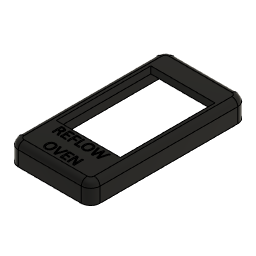
LCD Cover v3 (Autodesk Fusion 360 design; units mm, degrees)
Autodesk Fusion 360 part; units mm, degrees
(part 1 of 2)
sketch "Sketch1" plane through (0, 0, 0) normal (0, 0, 1) x (1, 0, 0)
  line L0 (27, -64) -> (-27, -64)
  line L1 (-32, -59) -> (-32, 59)
  line L2 (-27, 64) -> (27, 64)
  line L3 (32, 59) -> (32, -59)
  line L4 (32, -64) -> (-32, 64) construction
  line L5 (-32, -64) -> (32, 64) construction
  arc A0 (-27, 64) -> (-32, 59) centre (-27, 59) ccw
  arc A1 (32, 59) -> (27, 64) centre (27, 59) ccw
  arc A2 (-32, -59) -> (-27, -64) centre (-27, -59) ccw
  arc A3 (27, -64) -> (32, -59) centre (27, -59) ccw
  arc A4 (27, -67) -> (35, -59) centre (27, -59) ccw
  line L6 (35, 59) -> (35, -59)
  arc A5 (35, 59) -> (27, 67) centre (27, 59) ccw
  line L7 (-27, 67) -> (27, 67)
  arc A6 (-27, 67) -> (-35, 59) centre (-27, 59) ccw
  line L8 (-35, -59) -> (-35, 59)
  arc A7 (-35, -59) -> (-27, -67) centre (-27, -59) ccw
  line L9 (27, -67) -> (-27, -67)
  line L10 (24.75, 56.35) -> (-24.75, 56.35) construction
  line L11 (-24.75, 56.35) -> (-24.75, -37.75) construction
  line L12 (-24.75, -37.75) -> (24.75, -37.75) construction
  line L13 (24.75, -37.75) -> (24.75, 56.35) construction
  line L14 (24.75, 56.35) -> (-24.75, -37.75) construction
  line L15 (-24.75, 56.35) -> (24.75, -37.75) construction
  line L16 (0, 0) -> (0, 9.3) construction
  line L17 (24.48, 44) -> (-24.48, 44)
  line L18 (-24.48, 44) -> (-24.48, -31)
  line L19 (-24.48, -31) -> (24.48, -31)
  line L20 (24.48, -31) -> (24.48, 44)
  line L21 (24.48, 44) -> (-24.48, -31) construction
  line L22 (-24.48, 44) -> (24.48, -31) construction
  point P0 (0, 9.3)
  point P1 (0, 6.5)
  dimension "d1" = 64
  dimension "d2" = 128
  dimension "d3" = 5
  dimension "d4" = 5
  dimension "d5" = 5
  dimension "d6" = 5
  dimension "d7" = -3
  dimension "d8" = 49.5
  dimension "d9" = 94.1
  dimension "d11" = 54.7
  dimension "d12" = 48.96
  dimension "d13" = 75
  dimension "d14" = 12.35
  dimension "d24" = 15.56
  dimension "d25" = 39
  constraint horizontal L0
  constraint perpendicular L0 L1
  constraint parallel L0 L2
  constraint parallel L1 L3
  constraint coincident L4 L16.start
  constraint coincident L5 L16.start
  constraint coincident L16.start origin
  constraint coincident L4.end L1
  constraint coincident L4.end L2
  constraint tangent L1 A0
  constraint tangent L2 A0
  constraint coincident L5.end L2
  constraint coincident L5.end L3
  constraint tangent L2 A1
  constraint tangent L3 A1
  constraint coincident L5.start L1
  constraint coincident L5.start L0
  constraint tangent L1 A2
  constraint tangent L0 A2
  constraint coincident L4.start L0
  constraint coincident L4.start L3
  constraint tangent L0 A3
  constraint tangent L3 A3
  constraint horizontal L10
  constraint perpendicular L10 L11
  constraint parallel L10 L12
  constraint parallel L11 L13
  constraint coincident L14 P0
  constraint coincident L15 P0
  constraint coincident P0 L16.end
  constraint vertical L16
  constraint horizontal L17
  constraint perpendicular L17 L18
  constraint parallel L17 L19
  constraint parallel L18 L20
  constraint coincident L21 P1
  constraint coincident L22 P1
  constraint coincident L16 P1
  measures "d1" distance of L4.end L5.end
  measures "d2" distance of L5.start L4.end
  measures "d3" radius of A0
  measures "d4" radius of A1
  measures "d5" radius of A2
  measures "d6" radius of A3
  measures "d8" distance of L11.end L12.end
  measures "d9" distance of L10.end L11.end
  measures "d11" distance of L2 P0
  measures "d12" distance of L18.end L19.end
  measures "d13" distance of L17.end L18.end
  measures "d14" distance of L10 L17
extrude "Extrude1" add sketch "Sketch1" against normal blind 14.7 contours A4 L6 A5 L7 A6 L8 A7 L9
extrude "Extrude2" add sketch "Sketch1" along normal blind 3 contours L0 L1 L2 L3 A0 A1 A2 A3 | A4 L6 A5 L7 A6 L8 A7 L9
chamfer "Chamfer1" distance 3 angle 45 4 edges at (-24.48, 6.5, 3) (0, 44, 3) (24.48, 6.5, 3) (0, -31, 3)
fillet "Fillet1" radius 5 8 edges at (35, 0, 3) (32.6569, 64.6569, 3) (0, 67, 3) (-32.6569, 64.6569, 3) (-35, 0, 3) (-32.6569, -64.6569, 3) (0, -67, 3) (32.6569, -64.6569, 3)
fillet "Fillet2" radius 2 8 edges at (-32, 0, 0) (-30.5355, 62.5355, 0) (0, 64, 0) (30.5355, 62.5355, 0) (32, 0, 0) (30.5355, -62.5355, 0) (0, -64, 0) (-30.5355, -62.5355, 0)
sketch "Sketch2" plane through (0, 0, 3) normal (0, 0, 1) x (-1, 0, 0)
  line L0 (-27.48, -47) -> (-27.48, 34)
  line L1 (-27.48, 34) -> (27.48, 34)
  line L2 (27.48, 34) -> (27.48, -47)
  line L3 (27.48, -47) -> (-27.48, -47)
  line L4 (-30, 59) -> (-30, -59)
  arc A0 (-30, -59) -> (-27, -62) centre (-27, -59) ccw
  line L5 (-27, -62) -> (27, -62)
  arc A1 (27, -62) -> (30, -59) centre (27, -59) ccw
  line L6 (30, -59) -> (30, 59)
  arc A2 (30, 59) -> (27, 62) centre (27, 59) ccw
  line L7 (27, 62) -> (-27, 62)
  arc A3 (-27, 62) -> (-30, 59) centre (-27, 59) ccw
  line L8 (27.48, 34) -> (30, 34) construction
  line L9 (-27.48, 34) -> (-30, 34) construction
  line L10 (-30, 34) -> (29.1213, 61.1213) construction
  line L11 (30, 34) -> (-29.1213, 61.1213) construction
  line L12 (-1, 47.2622) -> (1, 47.2622) construction
  line L13 (1, 47.2622) -> (1, 48.2622) construction
  line L14 (1, 48.2622) -> (-1, 48.2622) construction
  line L15 (-1, 48.2622) -> (-1, 47.2622) construction
  line L16 (-1, 47.2622) -> (1, 48.2622) construction
  line L17 (1, 47.2622) -> (-1, 48.2622) construction
  spline S0 degree 3 poles (15.5846, 43.9099) (15.5852, 43.9255) (15.5864, 43.9553) (15.5977, 43.9829) (15.6031, 43.996) knots 0 0 0 0 0.004638 0.008871 0.008871 0.008871 0.008871
  spline S1 degree 3 poles (15.6031, 43.996) (15.6121, 44.0082) (15.6328, 44.0362) (15.6649, 44.0499) (15.6831, 44.0576) knots 0 0 0 0 0.004472 0.010255 0.010255 0.010255 0.010255
  spline S2 degree 3 poles (15.6831, 44.0576) (15.7075, 44.0655) (15.7637, 44.0836) (15.8223, 44.0906) (15.8554, 44.0945) knots 0 0 0 0 0.007692 0.017658 0.017658 0.017658 0.017658
  spline S3 degree 3 poles (15.8554, 44.0945) (15.8984, 44.0981) (15.9967, 44.1062) (16.0953, 44.1066) (16.1508, 44.1068) knots 0 0 0 0 0.012956 0.029574 0.029574 0.029574 0.029574
  spline S4 degree 3 poles (16.1508, 44.1068) (16.1993, 44.1066) (16.2866, 44.1061) (16.3736, 44.0981) (16.4123, 44.0945) knots 0 0 0 0 0.014542 0.026194 0.026194 0.026194 0.026194
  spline S5 degree 3 poles (16.4123, 44.0945) (16.4431, 44.0903) (16.499, 44.0828) (16.5517, 44.0633) (16.5754, 44.0545) knots 0 0 0 0 0.009295 0.016836 0.016836 0.016836 0.016836
  spline S6 degree 3 poles (16.5754, 44.0545) (16.5945, 44.0447) (16.6317, 44.0256) (16.658, 43.9932) (16.6708, 43.9776) knots 0 0 0 0 0.006385 0.012372 0.012372 0.012372 0.012372
  spline S7 degree 3 poles (16.6708, 43.9776) (16.6819, 43.9594) (16.7058, 43.9205) (16.7211, 43.8775) (16.7292, 43.8545) knots 0 0 0 0 0.006373 0.013658 0.013658 0.013658 0.013658
  line L18 (16.7292, 43.8545) -> (17.4615, 41.9776)
  spline S8 degree 3 poles (17.4615, 41.9776) (17.5042, 41.8747) (17.5866, 41.6757) (17.6828, 41.483) (17.7292, 41.3899) knots 0 0 0 0 0.033392 0.064596 0.064596 0.064596 0.064596
  spline S9 degree 3 poles (17.7292, 41.3899) (17.7767, 41.3046) (17.8692, 41.1384) (17.9965, 40.9972) (18.0585, 40.9284) knots 0 0 0 0 0.029168 0.056854 0.056854 0.056854 0.056854
  spline S10 degree 3 poles (18.0585, 40.9284) (18.1252, 40.8672) (18.2597, 40.744) (18.4246, 40.6661) (18.5077, 40.6268) knots 0 0 0 0 0.026986 0.05438 0.05438 0.05438 0.05438
  spline S11 degree 3 poles (18.5077, 40.6268) (18.6018, 40.5954) (18.8033, 40.5282) (19.0159, 40.5223) (19.1292, 40.5191) knots 0 0 0 0 0.029585 0.063385 0.063385 0.063385 0.063385
  line L19 (19.1292, 40.5191) -> (19.8369, 40.5191)
  line L20 (19.8369, 40.5191) -> (19.8369, 43.9099)
  spline S12 degree 3 poles (19.8369, 43.9099) (19.838, 43.9257) (19.8401, 43.9567) (19.8565, 43.9831) (19.8646, 43.996) knots 0 0 0 0 0.004667 0.009174 0.009174 0.009174 0.009174
  spline S13 degree 3 poles (19.8646, 43.996) (19.8758, 44.008) (19.9001, 44.0338) (19.933, 44.0473) (19.9508, 44.0545) knots 0 0 0 0 0.004844 0.01052 0.01052 0.01052 0.01052
  spline S14 degree 3 poles (19.9508, 44.0545) (19.9737, 44.0617) (20.0261, 44.078) (20.0803, 44.0866) (20.1108, 44.0914) knots 0 0 0 0 0.007206 0.01644 0.01644 0.01644 0.01644
  spline S15 degree 3 poles (20.1108, 44.0914) (20.1489, 44.0959) (20.2338, 44.1059) (20.3192, 44.1065) (20.3662, 44.1068) knots 0 0 0 0 0.01152 0.025602 0.025602 0.025602 0.025602
  spline S16 degree 3 poles (20.3662, 44.1068) (20.4131, 44.1065) (20.4986, 44.1059) (20.5834, 44.0959) (20.6215, 44.0914) knots 0 0 0 0 0.014082 0.025602 0.025602 0.025602 0.025602
  spline S17 degree 3 poles (20.6215, 44.0914) (20.6522, 44.0865) (20.7074, 44.0778) (20.7609, 44.0617) (20.7846, 44.0545) knots 0 0 0 0 0.009309 0.016737 0.016737 0.016737 0.016737
  spline S18 degree 3 poles (20.7846, 44.0545) (20.803, 44.0475) (20.8365, 44.0346) (20.8601, 44.008) (20.8708, 43.996) knots 0 0 0 0 0.005814 0.010547 0.010547 0.010547 0.010547
  spline S19 degree 3 poles (20.8708, 43.996) (20.8779, 43.983) (20.8927, 43.9562) (20.8945, 43.9256) (20.8954, 43.9099) knots 0 0 0 0 0.004406 0.009062 0.009062 0.009062 0.009062
  line L21 (20.8954, 43.9099) -> (20.8954, 36.5376)
  spline S20 degree 3 poles (20.8954, 36.5376) (20.8932, 36.4662) (20.8892, 36.3389) (20.8059, 36.244) (20.7692, 36.2022) knots 0 0 0 0 0.020627 0.03683 0.03683 0.03683 0.03683
  spline S21 degree 3 poles (20.7692, 36.2022) (20.7273, 36.1744) (20.6458, 36.1204) (20.5487, 36.1112) (20.5015, 36.1068) knots 0 0 0 0 0.014839 0.028813 0.028813 0.028813 0.028813
  line L22 (20.5015, 36.1068) -> (18.8092, 36.1068)
  spline S22 degree 3 poles (18.8092, 36.1068) (18.7171, 36.1072) (18.5498, 36.1078) (18.3828, 36.1177) (18.3077, 36.1222) knots 0 0 0 0 0.027618 0.050186 0.050186 0.050186 0.050186
  spline S23 degree 3 poles (18.3077, 36.1222) (18.2443, 36.1273) (18.1242, 36.1369) (18.0043, 36.1499) (17.9477, 36.156) knots 0 0 0 0 0.019068 0.03616 0.03616 0.03616 0.03616
  spline S24 degree 3 poles (17.9477, 36.156) (17.8012, 36.1852) (17.5205, 36.241) (17.2579, 36.3542) (17.1323, 36.4084) knots 0 0 0 0 0.044667 0.085564 0.085564 0.085564 0.085564
  spline S25 degree 3 poles (17.1323, 36.4084) (17.0202, 36.4685) (16.8013, 36.5858) (16.6246, 36.7602) (16.5385, 36.8453) knots 0 0 0 0 0.037954 0.074067 0.074067 0.074067 0.074067
  spline S26 degree 3 poles (16.5385, 36.8453) (16.4634, 36.9369) (16.3127, 37.1207) (16.2233, 37.3409) (16.1785, 37.4514) knots 0 0 0 0 0.035308 0.070859 0.070859 0.070859 0.070859
  spline S27 degree 3 poles (16.1785, 37.4514) (16.1435, 37.5704) (16.0711, 37.8164) (16.0628, 38.0728) (16.0585, 38.2053) knots 0 0 0 0 0.037033 0.076609 0.076609 0.076609 0.076609
  spline S28 degree 3 poles (16.0585, 38.2053) (16.0621, 38.3325) (16.069, 38.576) (16.1348, 38.8103) (16.1662, 38.9222) knots 0 0 0 0 0.038018 0.07274 0.07274 0.07274 0.07274
  spline S29 degree 3 poles (16.1662, 38.9222) (16.2055, 39.0242) (16.2832, 39.2253) (16.413, 39.3974) (16.4769, 39.4822) knots 0 0 0 0 0.032616 0.064322 0.064322 0.064322 0.064322
  spline S30 degree 3 poles (16.4769, 39.4822) (16.5486, 39.5609) (16.694, 39.7206) (16.8725, 39.8421) (16.9631, 39.9037) knots 0 0 0 0 0.031821 0.064545 0.064545 0.064545 0.064545
  spline S31 degree 3 poles (16.9631, 39.9037) (17.0617, 39.9614) (17.2644, 40.08) (17.4841, 40.1628) (17.5969, 40.2053) knots 0 0 0 0 0.03422 0.070303 0.070303 0.070303 0.070303
  spline S32 degree 3 poles (17.5969, 40.2053) (17.5331, 40.2357) (17.4064, 40.2961) (17.2952, 40.3814) (17.24, 40.4237) knots 0 0 0 0 0.021159 0.04195 0.04195 0.04195 0.04195
  spline S33 degree 3 poles (17.24, 40.4237) (17.187, 40.4708) (17.078, 40.5675) (16.9878, 40.6819) (16.9415, 40.7407) knots 0 0 0 0 0.021223 0.04361 0.04361 0.04361 0.04361
  spline S34 degree 3 poles (16.9415, 40.7407) (16.8953, 40.806) (16.799, 40.9419) (16.7207, 41.0889) (16.68, 41.1653) knots 0 0 0 0 0.023981 0.049914 0.049914 0.049914 0.049914
  spline S35 degree 3 poles (16.68, 41.1653) (16.6381, 41.25) (16.5501, 41.4278) (16.4738, 41.611) (16.4338, 41.7068) knots 0 0 0 0 0.028349 0.059499 0.059499 0.059499 0.059499
  line L23 (16.4338, 41.7068) -> (15.72, 43.4607)
  spline S36 degree 3 poles (15.72, 43.4607) (15.6956, 43.5232) (15.6555, 43.6257) (15.6222, 43.7305) (15.6092, 43.7714) knots 0 0 0 0 0.020131 0.032999 0.032999 0.032999 0.032999
  spline S37 degree 3 poles (15.6092, 43.7714) (15.6021, 43.7977) (15.5898, 43.8431) (15.5861, 43.8901) (15.5846, 43.9099) knots 0 0 0 0 0.008135 0.01409 0.01409 0.01409 0.01409
  spline S38 degree 3 poles (17.1785, 38.3161) (17.1852, 38.1693) (17.1981, 37.8902) (17.3267, 37.6427) (17.3877, 37.5253) knots 0 0 0 0 0.04347 0.082671 0.082671 0.082671 0.082671
  spline S39 degree 3 poles (17.3877, 37.5253) (17.4748, 37.4237) (17.6639, 37.2032) (17.9403, 37.1106) (18.0892, 37.0607) knots 0 0 0 0 0.039435 0.085547 0.085547 0.085547 0.085547
  spline S40 degree 3 poles (18.0892, 37.0607) (18.1436, 37.0472) (18.2581, 37.0189) (18.3754, 37.0059) (18.4369, 36.9991) knots 0 0 0 0 0.016795 0.035344 0.035344 0.035344 0.035344
  spline S41 degree 3 poles (18.4369, 36.9991) (18.5115, 36.9938) (18.6805, 36.9816) (18.85, 36.981) (18.9446, 36.9807) knots 0 0 0 0 0.022427 0.050816 0.050816 0.050816 0.050816
  line L24 (18.9446, 36.9807) -> (19.8369, 36.9807)
  line L25 (19.8369, 36.9807) -> (19.8369, 39.6637)
  line L26 (19.8369, 39.6637) -> (18.8031, 39.6637)
  spline S42 degree 3 poles (18.8031, 39.6637) (18.6723, 39.6608) (18.4271, 39.6552) (18.1904, 39.5918) (18.08, 39.5622) knots 0 0 0 0 0.039082 0.07325 0.07325 0.07325 0.07325
  spline S43 degree 3 poles (18.08, 39.5622) (17.9843, 39.5264) (17.8006, 39.4577) (17.6462, 39.337) (17.5723, 39.2791) knots 0 0 0 0 0.030454 0.058434 0.058434 0.058434 0.058434
  spline S44 degree 3 poles (17.5723, 39.2791) (17.5092, 39.2163) (17.3841, 39.0916) (17.3104, 38.931) (17.2738, 38.8514) knots 0 0 0 0 0.026479 0.052529 0.052529 0.052529 0.052529
  spline S45 degree 3 poles (17.2738, 38.8514) (17.246, 38.7665) (17.1891, 38.5926) (17.182, 38.4097) (17.1785, 38.3161) knots 0 0 0 0 0.02667 0.054618 0.054618 0.054618 0.054618
  spline S46 degree 3 poles (9.6215, 43.633) (9.6219, 43.6676) (9.6226, 43.7325) (9.6303, 43.7969) (9.6338, 43.8268) knots 0 0 0 0 0.010389 0.019436 0.019436 0.019436 0.019436
  spline S47 degree 3 poles (9.6338, 43.8268) (9.6383, 43.8526) (9.6466, 43.9007) (9.6673, 43.9448) (9.6769, 43.9653) knots 0 0 0 0 0.007801 0.014559 0.014559 0.014559 0.014559
  spline S48 degree 3 poles (9.6769, 43.9653) (9.687, 43.9821) (9.7056, 44.0132) (9.7344, 44.0352) (9.7477, 44.0453) knots 0 0 0 0 0.005804 0.010768 0.010768 0.010768 0.010768
  spline S49 degree 3 poles (9.7477, 44.0453) (9.7615, 44.0525) (9.7895, 44.067) (9.821, 44.0689) (9.8369, 44.0699) knots 0 0 0 0 0.004616 0.009348 0.009348 0.009348 0.009348
  line L27 (9.8369, 44.0699) -> (13.6585, 44.0699)
  spline S50 degree 3 poles (13.6585, 44.0699) (13.7056, 44.0655) (13.8028, 44.0563) (13.8842, 44.0023) (13.9262, 43.9745) knots 0 0 0 0 0.013974 0.028813 0.028813 0.028813 0.028813
  spline S51 degree 3 poles (13.9262, 43.9745) (13.9628, 43.9328) (14.0461, 43.8379) (14.0501, 43.7105) (14.0523, 43.6391) knots 0 0 0 0 0.016203 0.03683 0.03683 0.03683 0.03683
  line L28 (14.0523, 43.6391) -> (14.0523, 36.5376)
  spline S52 degree 3 poles (14.0523, 36.5376) (14.0501, 36.4662) (14.0461, 36.3389) (13.9628, 36.244) (13.9262, 36.2022) knots 0 0 0 0 0.020627 0.03683 0.03683 0.03683 0.03683
  spline S53 degree 3 poles (13.9262, 36.2022) (13.8842, 36.1744) (13.8028, 36.1204) (13.7056, 36.1112) (13.6585, 36.1068) knots 0 0 0 0 0.014838 0.028813 0.028813 0.028813 0.028813
  line L29 (13.6585, 36.1068) -> (9.88, 36.1068)
  spline S54 degree 3 poles (9.88, 36.1068) (9.8641, 36.1078) (9.8326, 36.1097) (9.8046, 36.1243) (9.7908, 36.1314) knots 0 0 0 0 0.004732 0.009349 0.009349 0.009349 0.009349
  spline S55 degree 3 poles (9.7908, 36.1314) (9.7778, 36.1415) (9.7501, 36.163) (9.7345, 36.1946) (9.7262, 36.2114) knots 0 0 0 0 0.004849 0.010403 0.010403 0.010403 0.010403
  spline S56 degree 3 poles (9.7262, 36.2114) (9.7182, 36.232) (9.7007, 36.277) (9.6913, 36.3243) (9.6862, 36.3499) knots 0 0 0 0 0.006618 0.014436 0.014436 0.014436 0.014436
  spline S57 degree 3 poles (9.6862, 36.3499) (9.6817, 36.3809) (9.6718, 36.4492) (9.6711, 36.5183) (9.6708, 36.556) knots 0 0 0 0 0.009379 0.020693 0.020693 0.020693 0.020693
  spline S58 degree 3 poles (9.6708, 36.556) (9.6712, 36.5907) (9.6721, 36.6557) (9.6817, 36.7199) (9.6862, 36.7499) knots 0 0 0 0 0.010392 0.019465 0.019465 0.019465 0.019465
  spline S59 degree 3 poles (9.6862, 36.7499) (9.6912, 36.7753) (9.7004, 36.8216) (9.7181, 36.8655) (9.7262, 36.8853) knots 0 0 0 0 0.007743 0.014145 0.014145 0.014145 0.014145
  spline S60 degree 3 poles (9.7262, 36.8853) (9.7346, 36.9013) (9.7506, 36.9317) (9.7779, 36.9524) (9.7908, 36.9622) knots 0 0 0 0 0.005357 0.010155 0.010155 0.010155 0.010155
  spline S61 degree 3 poles (9.7908, 36.9622) (9.8046, 36.9694) (9.8326, 36.9839) (9.8641, 36.9858) (9.88, 36.9868) knots 0 0 0 0 0.004616 0.009349 0.009349 0.009349 0.009349
  line L30 (9.88, 36.9868) -> (12.9938, 36.9868)
  line L31 (12.9938, 36.9868) -> (12.9938, 39.4853)
  line L32 (12.9938, 39.4853) -> (10.3231, 39.4853)
  spline S62 degree 3 poles (10.3231, 39.4853) (10.3071, 39.4864) (10.2752, 39.4887) (10.2476, 39.5049) (10.2338, 39.513) knots 0 0 0 0 0.004743 0.009456 0.009456 0.009456 0.009456
  spline S63 degree 3 poles (10.2338, 39.513) (10.2209, 39.5234) (10.1938, 39.5451) (10.1756, 39.5746) (10.1662, 39.5899) knots 0 0 0 0 0.004957 0.010314 0.010314 0.010314 0.010314
  spline S64 degree 3 poles (10.1662, 39.5899) (10.1574, 39.6091) (10.1377, 39.6523) (10.1303, 39.6993) (10.1262, 39.7253) knots 0 0 0 0 0.006314 0.014174 0.014174 0.014174 0.014174
  spline S65 degree 3 poles (10.1262, 39.7253) (10.1226, 39.7565) (10.1148, 39.824) (10.1142, 39.8919) (10.1138, 39.9284) knots 0 0 0 0 0.00943 0.020357 0.020357 0.020357 0.020357
  spline S66 degree 3 poles (10.1138, 39.9284) (10.1142, 39.9628) (10.1148, 40.0266) (10.1226, 40.0899) (10.1262, 40.1191) knots 0 0 0 0 0.010312 0.01913 0.01913 0.01913 0.01913
  spline S67 degree 3 poles (10.1262, 40.1191) (10.1304, 40.1436) (10.1382, 40.1884) (10.1574, 40.2296) (10.1662, 40.2484) knots 0 0 0 0 0.007409 0.013581 0.013581 0.013581 0.013581
  spline S68 degree 3 poles (10.1662, 40.2484) (10.1755, 40.2634) (10.1931, 40.2918) (10.2208, 40.3104) (10.2338, 40.3191) knots 0 0 0 0 0.005231 0.009893 0.009893 0.009893 0.009893
  spline S69 degree 3 poles (10.2338, 40.3191) (10.2477, 40.3254) (10.2761, 40.3382) (10.3072, 40.3398) (10.3231, 40.3407) knots 0 0 0 0 0.004529 0.009252 0.009252 0.009252 0.009252
  line L33 (10.3231, 40.3407) -> (12.9938, 40.3407)
  line L34 (12.9938, 40.3407) -> (12.9938, 43.1899)
  line L35 (12.9938, 43.1899) -> (9.8369, 43.1899)
  spline S70 degree 3 poles (9.8369, 43.1899) (9.821, 43.1909) (9.7895, 43.1928) (9.7615, 43.2073) (9.7477, 43.2145) knots 0 0 0 0 0.004732 0.009348 0.009348 0.009348 0.009348
  spline S71 degree 3 poles (9.7477, 43.2145) (9.7344, 43.2244) (9.7061, 43.2456) (9.6871, 43.2755) (9.6769, 43.2914) knots 0 0 0 0 0.004915 0.010531 0.010531 0.010531 0.010531
  spline S72 degree 3 poles (9.6769, 43.2914) (9.6673, 43.3111) (9.6463, 43.3541) (9.6382, 43.4013) (9.6338, 43.4268) knots 0 0 0 0 0.006545 0.014271 0.014271 0.014271 0.014271
  spline S73 degree 3 poles (9.6338, 43.4268) (9.6303, 43.4578) (9.6223, 43.5263) (9.6218, 43.5952) (9.6215, 43.633) knots 0 0 0 0 0.009353 0.020665 0.020665 0.020665 0.020665
  spline S74 degree 3 poles (3.7138, 36.5622) (3.7142, 36.5987) (3.7148, 36.6666) (3.7226, 36.734) (3.7262, 36.7653) knots 0 0 0 0 0.010927 0.020357 0.020357 0.020357 0.020357
  spline S75 degree 3 poles (3.7262, 36.7653) (3.7305, 36.7916) (3.7384, 36.8398) (3.7596, 36.8838) (3.7692, 36.9037) knots 0 0 0 0 0.007951 0.014567 0.014567 0.014567 0.014567
  spline S76 degree 3 poles (3.7692, 36.9037) (3.7794, 36.9197) (3.7984, 36.9496) (3.8268, 36.9708) (3.84, 36.9807) knots 0 0 0 0 0.005616 0.010531 0.010531 0.010531 0.010531
  spline S77 degree 3 poles (3.84, 36.9807) (3.8533, 36.9878) (3.8793, 37.0019) (3.9087, 37.0042) (3.9231, 37.0053) knots 0 0 0 0 0.004475 0.008751 0.008751 0.008751 0.008751
  line L36 (3.9231, 37.0053) -> (6.84, 37.0053)
  line L37 (6.84, 37.0053) -> (6.84, 39.713)
  line L38 (6.84, 39.713) -> (4.0831, 39.713)
  spline S78 degree 3 poles (4.0831, 39.713) (4.0688, 39.7139) (4.0397, 39.7158) (4.0134, 39.7282) (4, 39.7345) knots 0 0 0 0 0.004265 0.00865 0.00865 0.00865 0.00865
  spline S79 degree 3 poles (4, 39.7345) (3.9868, 39.7433) (3.9585, 39.7621) (3.9394, 39.7903) (3.9292, 39.8053) knots 0 0 0 0 0.004723 0.010093 0.010093 0.010093 0.010093
  spline S80 degree 3 poles (3.9292, 39.8053) (3.9196, 39.8242) (3.8983, 39.866) (3.8905, 39.9123) (3.8862, 39.9376) knots 0 0 0 0 0.006334 0.013985 0.013985 0.013985 0.013985
  spline S81 degree 3 poles (3.8862, 39.9376) (3.8826, 39.9691) (3.8746, 40.0396) (3.8741, 40.1106) (3.8738, 40.1499) knots 0 0 0 0 0.009506 0.02128 0.02128 0.02128 0.02128
  spline S82 degree 3 poles (3.8738, 40.1499) (3.8742, 40.1861) (3.8748, 40.253) (3.8826, 40.3194) (3.8862, 40.3499) knots 0 0 0 0 0.010851 0.020051 0.020051 0.020051 0.020051
  spline S83 degree 3 poles (3.8862, 40.3499) (3.8905, 40.3754) (3.8986, 40.4226) (3.9196, 40.4656) (3.9292, 40.4853) knots 0 0 0 0 0.007726 0.014271 0.014271 0.014271 0.014271
  spline S84 degree 3 poles (3.9292, 40.4853) (3.9394, 40.5014) (3.9588, 40.5319) (3.9868, 40.5546) (4, 40.5653) knots 0 0 0 0 0.005678 0.010744 0.010744 0.010744 0.010744
  spline S85 degree 3 poles (4, 40.5653) (4.0132, 40.5734) (4.0388, 40.589) (4.0686, 40.5917) (4.0831, 40.593) knots 0 0 0 0 0.004575 0.008863 0.008863 0.008863 0.008863
  line L39 (4.0831, 40.593) -> (6.84, 40.593)
  line L40 (6.84, 40.593) -> (6.84, 43.9099)
  spline S86 degree 3 poles (6.84, 43.9099) (6.8411, 43.9243) (6.8434, 43.9537) (6.8574, 43.9797) (6.8646, 43.993) knots 0 0 0 0 0.004275 0.008751 0.008751 0.008751 0.008751
  spline S87 degree 3 poles (6.8646, 43.993) (6.8751, 44.0058) (6.8982, 44.0339) (6.9323, 44.0473) (6.9508, 44.0545) knots 0 0 0 0 0.004897 0.010745 0.010745 0.010745 0.010745
  spline S88 degree 3 poles (6.9508, 44.0545) (6.9742, 44.0616) (7.0267, 44.0776) (7.0809, 44.0865) (7.1108, 44.0914) knots 0 0 0 0 0.007354 0.016436 0.016436 0.016436 0.016436
  spline S89 degree 3 poles (7.1108, 44.0914) (7.1487, 44.0959) (7.2345, 44.106) (7.321, 44.1065) (7.3692, 44.1068) knots 0 0 0 0 0.011443 0.02591 0.02591 0.02591 0.02591
  spline S90 degree 3 poles (7.3692, 44.1068) (7.4149, 44.1064) (7.4993, 44.1057) (7.5831, 44.0959) (7.6215, 44.0914) knots 0 0 0 0 0.013698 0.025294 0.025294 0.025294 0.025294
  spline S91 degree 3 poles (7.6215, 44.0914) (7.653, 44.0866) (7.7092, 44.0779) (7.7637, 44.0617) (7.7877, 44.0545) knots 0 0 0 0 0.009536 0.017038 0.017038 0.017038 0.017038
  spline S92 degree 3 poles (7.7877, 44.0545) (7.8062, 44.0473) (7.8402, 44.0339) (7.8633, 44.0058) (7.8738, 43.993) knots 0 0 0 0 0.005848 0.010745 0.010745 0.010745 0.010745
  spline S93 degree 3 poles (7.8738, 43.993) (7.881, 43.9797) (7.8951, 43.9537) (7.8973, 43.9243) (7.8985, 43.9099) knots 0 0 0 0 0.004475 0.008751 0.008751 0.008751 0.008751
  line L41 (7.8985, 43.9099) -> (7.8985, 36.5376)
  spline S94 degree 3 poles (7.8985, 36.5376) (7.8962, 36.4662) (7.8923, 36.3389) (7.809, 36.244) (7.7723, 36.2022) knots 0 0 0 0 0.020627 0.03683 0.03683 0.03683 0.03683
  spline S95 degree 3 poles (7.7723, 36.2022) (7.7304, 36.1744) (7.6489, 36.1204) (7.5517, 36.1112) (7.5046, 36.1068) knots 0 0 0 0 0.014838 0.028813 0.028813 0.028813 0.028813
  line L42 (7.5046, 36.1068) -> (3.9231, 36.1068)
  spline S96 degree 3 poles (3.9231, 36.1068) (3.9087, 36.1079) (3.8793, 36.1102) (3.8533, 36.1243) (3.84, 36.1314) knots 0 0 0 0 0.004275 0.008751 0.008751 0.008751 0.008751
  spline S97 degree 3 poles (3.84, 36.1314) (3.8267, 36.1416) (3.7979, 36.1635) (3.7793, 36.1946) (3.7692, 36.2114) knots 0 0 0 0 0.004964 0.010768 0.010768 0.010768 0.010768
  spline S98 degree 3 poles (3.7692, 36.2114) (3.7596, 36.2324) (3.7385, 36.2786) (3.7305, 36.3287) (3.7262, 36.356) knots 0 0 0 0 0.0069 0.015152 0.015152 0.015152 0.015152
  spline S99 degree 3 poles (3.7262, 36.356) (3.7226, 36.3881) (3.7149, 36.4566) (3.7142, 36.5255) (3.7138, 36.5622) knots 0 0 0 0 0.00966 0.020664 0.020664 0.020664 0.020664
  spline S100 degree 3 poles (-2.0215, 43.6084) (-2.0213, 43.6461) (-2.0207, 43.715) (-2.0128, 43.7835) (-2.0092, 43.8145) knots 0 0 0 0 0.011312 0.020665 0.020665 0.020665 0.020665
  spline S101 degree 3 poles (-2.0092, 43.8145) (-2.0048, 43.8404) (-1.9966, 43.8891) (-1.9779, 43.9347) (-1.9692, 43.956) knots 0 0 0 0 0.00786 0.014748 0.014748 0.014748 0.014748
  spline S102 degree 3 poles (-1.9692, 43.956) (-1.9601, 43.9738) (-1.943, 44.007) (-1.9146, 44.0311) (-1.9015, 44.0422) knots 0 0 0 0 0.005937 0.011051 0.011051 0.011051 0.011051
  spline S103 degree 3 poles (-1.9015, 44.0422) (-1.8873, 44.0503) (-1.8577, 44.067) (-1.8237, 44.0689) (-1.8062, 44.0699) knots 0 0 0 0 0.004852 0.010052 0.010052 0.010052 0.010052
  line L43 (-1.8062, 44.0699) -> (1.7138, 44.0699)
  spline S104 degree 3 poles (1.7138, 44.0699) (1.761, 44.0655) (1.8582, 44.0563) (1.9396, 44.0023) (1.9815, 43.9745) knots 0 0 0 0 0.013974 0.028813 0.028813 0.028813 0.028813
  spline S105 degree 3 poles (1.9815, 43.9745) (2.0182, 43.9328) (2.1015, 43.8379) (2.1055, 43.7105) (2.1077, 43.6391) knots 0 0 0 0 0.016203 0.03683 0.03683 0.03683 0.03683
  line L44 (2.1077, 43.6391) -> (2.1077, 36.2668)
  spline S106 degree 3 poles (2.1077, 36.2668) (2.1068, 36.2511) (2.105, 36.2205) (2.0903, 36.1937) (2.0831, 36.1807) knots 0 0 0 0 0.004656 0.009062 0.009062 0.009062 0.009062
  spline S107 degree 3 poles (2.0831, 36.1807) (2.0724, 36.1687) (2.0488, 36.1421) (2.0153, 36.1293) (1.9969, 36.1222) knots 0 0 0 0 0.004732 0.010547 0.010547 0.010547 0.010547
  spline S108 degree 3 poles (1.9969, 36.1222) (1.9729, 36.115) (1.9184, 36.0988) (1.8622, 36.0901) (1.8308, 36.0853) knots 0 0 0 0 0.007502 0.017038 0.017038 0.017038 0.017038
  spline S109 degree 3 poles (1.8308, 36.0853) (1.7923, 36.0808) (1.7085, 36.071) (1.6242, 36.0703) (1.5785, 36.0699) knots 0 0 0 0 0.011596 0.025294 0.025294 0.025294 0.025294
  spline S110 degree 3 poles (1.5785, 36.0699) (1.5315, 36.0702) (1.4461, 36.0709) (1.3612, 36.0808) (1.3231, 36.0853) knots 0 0 0 0 0.014082 0.025602 0.025602 0.025602 0.025602
  spline S111 degree 3 poles (1.3231, 36.0853) (1.2924, 36.0902) (1.2372, 36.099) (1.1837, 36.1151) (1.16, 36.1222) knots 0 0 0 0 0.009309 0.016737 0.016737 0.016737 0.016737
  spline S112 degree 3 poles (1.16, 36.1222) (1.1416, 36.1293) (1.1082, 36.1421) (1.0845, 36.1687) (1.0738, 36.1807) knots 0 0 0 0 0.005814 0.010547 0.010547 0.010547 0.010547
  spline S113 degree 3 poles (1.0738, 36.1807) (1.0667, 36.1937) (1.0519, 36.2205) (1.0501, 36.2511) (1.0492, 36.2668) knots 0 0 0 0 0.004406 0.009062 0.009062 0.009062 0.009062
  line L45 (1.0492, 36.2668) -> (1.0492, 43.153)
  line L46 (1.0492, 43.153) -> (-1.8062, 43.153)
  spline S114 degree 3 poles (-1.8062, 43.153) (-1.8237, 43.154) (-1.8577, 43.1559) (-1.8873, 43.1726) (-1.9015, 43.1807) knots 0 0 0 0 0.0052 0.010052 0.010052 0.010052 0.010052
  spline S115 degree 3 poles (-1.9015, 43.1807) (-1.9146, 43.1913) (-1.942, 43.2138) (-1.9599, 43.2445) (-1.9692, 43.2607) knots 0 0 0 0 0.005009 0.010556 0.010556 0.010556 0.010556
  spline S116 degree 3 poles (-1.9692, 43.2607) (-1.978, 43.2807) (-1.9973, 43.325) (-2.005, 43.3729) (-2.0092, 43.3991) knots 0 0 0 0 0.006528 0.014463 0.014463 0.014463 0.014463
  spline S117 degree 3 poles (-2.0092, 43.3991) (-2.0128, 43.4309) (-2.0207, 43.5004) (-2.0212, 43.5704) (-2.0215, 43.6084) knots 0 0 0 0 0.009583 0.020972 0.020972 0.020972 0.020972
  spline S118 degree 3 poles (-9.5846, 39.996) (-9.577, 40.3037) (-9.5623, 40.8924) (-9.4233, 41.4645) (-9.3569, 41.7376) knots 0 0 0 0 0.092022 0.176083 0.176083 0.176083 0.176083
  spline S119 degree 3 poles (-9.3569, 41.7376) (-9.2744, 41.9831) (-9.1148, 42.4579) (-8.8195, 42.8623) (-8.6769, 43.0576) knots 0 0 0 0 0.077178 0.149269 0.149269 0.149269 0.149269
  spline S120 degree 3 poles (-8.6769, 43.0576) (-8.5151, 43.2292) (-8.1874, 43.5768) (-7.7586, 43.7877) (-7.5415, 43.8945) knots 0 0 0 0 0.070141 0.142072 0.142072 0.142072 0.142072
  spline S121 degree 3 poles (-7.5415, 43.8945) (-7.2972, 43.9797) (-6.7814, 44.1595) (-6.2351, 44.1774) (-5.9477, 44.1868) knots 0 0 0 0 0.077179 0.162876 0.162876 0.162876 0.162876
  spline S122 degree 3 poles (-5.9477, 44.1868) (-5.6659, 44.1787) (-5.1348, 44.1633) (-4.6306, 43.9971) (-4.3938, 43.9191) knots 0 0 0 0 0.084036 0.158412 0.158412 0.158412 0.158412
  spline S123 degree 3 poles (-4.3938, 43.9191) (-4.186, 43.8212) (-3.7769, 43.6283) (-3.4645, 43.3015) (-3.3108, 43.1407) knots 0 0 0 0 0.068267 0.1344 0.1344 0.1344 0.1344
  spline S124 degree 3 poles (-3.3108, 43.1407) (-3.176, 42.9552) (-2.8944, 42.5678) (-2.7494, 42.1111) (-2.6738, 41.873) knots 0 0 0 0 0.068317 0.142693 0.142693 0.142693 0.142693
  spline S125 degree 3 poles (-2.6738, 41.873) (-2.6129, 41.6028) (-2.4836, 41.0296) (-2.4712, 40.442) (-2.4646, 40.1314) knots 0 0 0 0 0.082884 0.1758 0.1758 0.1758 0.1758
  spline S126 degree 3 poles (-2.4646, 40.1314) (-2.4725, 39.8304) (-2.4876, 39.2519) (-2.6259, 38.6901) (-2.6923, 38.4207) knots 0 0 0 0 0.090026 0.173033 0.173033 0.173033 0.173033
  spline S127 degree 3 poles (-2.6923, 38.4207) (-2.775, 38.1771) (-2.9351, 37.7056) (-3.2319, 37.3061) (-3.3754, 37.113) knots 0 0 0 0 0.076635 0.148341 0.148341 0.148341 0.148341
  spline S128 degree 3 poles (-3.3754, 37.113) (-3.5382, 36.9431) (-3.8682, 36.5987) (-4.2967, 36.3886) (-4.5138, 36.2822) knots 0 0 0 0 0.069994 0.141916 0.141916 0.141916 0.141916
  spline S129 degree 3 poles (-4.5138, 36.2822) (-4.7582, 36.197) (-5.274, 36.0172) (-5.8203, 35.9993) (-6.1077, 35.9899) knots 0 0 0 0 0.077179 0.162876 0.162876 0.162876 0.162876
  spline S130 degree 3 poles (-6.1077, 35.9899) (-6.3845, 35.9982) (-6.9082, 36.0138) (-7.4055, 36.1774) (-7.64, 36.2545) knots 0 0 0 0 0.082573 0.156221 0.156221 0.156221 0.156221
  spline S131 degree 3 poles (-7.64, 36.2545) (-7.8473, 36.3517) (-8.2563, 36.5433) (-8.571, 36.8671) (-8.7262, 37.0268) knots 0 0 0 0 0.068052 0.134259 0.134259 0.134259 0.134259
  spline S132 degree 3 poles (-8.7262, 37.0268) (-8.8628, 37.2106) (-9.1472, 37.5931) (-9.2953, 38.0466) (-9.3723, 38.2822) knots 0 0 0 0 0.068228 0.142024 0.142024 0.142024 0.142024
  spline S133 degree 3 poles (-9.3723, 38.2822) (-9.4342, 38.5485) (-9.5651, 39.1121) (-9.5779, 39.6908) (-9.5846, 39.996) knots 0 0 0 0 0.081796 0.173104 0.173104 0.173104 0.173104
  spline S134 degree 3 poles (-8.4646, 40.0699) (-8.4603, 39.8517) (-8.452, 39.4291) (-8.3797, 39.0127) (-8.3448, 38.8114) knots 0 0 0 0 0.065376 0.126579 0.126579 0.126579 0.126579
  spline S135 degree 3 poles (-8.3448, 38.8114) (-8.3001, 38.627) (-8.214, 38.2717) (-8.0325, 37.9546) (-7.9452, 37.8022) knots 0 0 0 0 0.05661 0.109028 0.109028 0.109028 0.109028
  spline S136 degree 3 poles (-7.9452, 37.8022) (-7.8437, 37.6672) (-7.639, 37.3952) (-7.3461, 37.2218) (-7.1985, 37.1345) knots 0 0 0 0 0.05016 0.101042 0.101042 0.101042 0.101042
  spline S137 degree 3 poles (-7.1985, 37.1345) (-7.0265, 37.0646) (-6.6566, 36.9142) (-6.2569, 36.9014) (-6.0431, 36.8945) knots 0 0 0 0 0.055253 0.118841 0.118841 0.118841 0.118841
  spline S138 degree 3 poles (-6.0431, 36.8945) (-5.8288, 36.9021) (-5.4269, 36.9164) (-5.0593, 37.0777) (-4.8876, 37.153) knots 0 0 0 0 0.063634 0.119357 0.119357 0.119357 0.119357
  spline S139 degree 3 poles (-4.8876, 37.153) (-4.7395, 37.2458) (-4.4453, 37.4303) (-4.2337, 37.7055) (-4.1286, 37.8422) knots 0 0 0 0 0.051973 0.103258 0.103258 0.103258 0.103258
  spline S140 degree 3 poles (-4.1286, 37.8422) (-4.0376, 37.9947) (-3.8496, 38.3097) (-3.7579, 38.665) (-3.7106, 38.8484) knots 0 0 0 0 0.052985 0.109449 0.109449 0.109449 0.109449
  spline S141 degree 3 poles (-3.7106, 38.8484) (-3.6739, 39.0445) (-3.599, 39.4441) (-3.5895, 39.8506) (-3.5846, 40.0576) knots 0 0 0 0 0.059752 0.121755 0.121755 0.121755 0.121755
  spline S142 degree 3 poles (-3.5846, 40.0576) (-3.5887, 40.2827) (-3.5965, 40.7164) (-3.6673, 41.1442) (-3.7014, 41.3499) knots 0 0 0 0 0.067448 0.129911 0.129911 0.129911 0.129911
  spline S143 degree 3 poles (-3.7014, 41.3499) (-3.7449, 41.5367) (-3.8282, 41.8948) (-4.0085, 42.2151) (-4.0948, 42.3684) knots 0 0 0 0 0.05719 0.109673 0.109673 0.109673 0.109673
  spline S144 degree 3 poles (-4.0948, 42.3684) (-4.1952, 42.5032) (-4.3974, 42.7745) (-4.6888, 42.9465) (-4.8354, 43.033) knots 0 0 0 0 0.049902 0.100404 0.100404 0.100404 0.100404
  spline S145 degree 3 poles (-4.8354, 43.033) (-5.0077, 43.102) (-5.3809, 43.2514) (-5.7834, 43.2634) (-6, 43.2699) knots 0 0 0 0 0.055253 0.11967 0.11967 0.11967 0.11967
  spline S146 degree 3 poles (-6, 43.2699) (-6.2163, 43.2623) (-6.6221, 43.248) (-6.9941, 43.0867) (-7.1678, 43.0114) knots 0 0 0 0 0.064246 0.120547 0.120547 0.120547 0.120547
  spline S147 degree 3 poles (-7.1678, 43.0114) (-7.3176, 42.9182) (-7.6152, 42.7329) (-7.8254, 42.4523) (-7.9299, 42.313) knots 0 0 0 0 0.05242 0.104181 0.104181 0.104181 0.104181
  spline S148 degree 3 poles (-7.9299, 42.313) (-8.0198, 42.1578) (-8.2052, 41.8379) (-8.2953, 41.4792) (-8.3417, 41.2945) knots 0 0 0 0 0.053521 0.110337 0.110337 0.110337 0.110337
  spline S149 degree 3 poles (-8.3417, 41.2945) (-8.3775, 41.0966) (-8.4509, 40.6917) (-8.46, 40.2802) (-8.4646, 40.0699) knots 0 0 0 0 0.060248 0.123246 0.123246 0.123246 0.123246
  spline S150 degree 3 poles (-18.7477, 43.836) (-18.739, 43.8628) (-18.7225, 43.9134) (-18.6894, 43.9549) (-18.6739, 43.9745) knots 0 0 0 0 0.008356 0.015805 0.015805 0.015805 0.015805
  spline S151 degree 3 poles (-18.6739, 43.9745) (-18.6551, 43.9912) (-18.6153, 44.0266) (-18.5651, 44.0448) (-18.5385, 44.0545) knots 0 0 0 0 0.007449 0.015853 0.015853 0.015853 0.015853
  spline S152 degree 3 poles (-18.5385, 44.0545) (-18.5066, 44.0632) (-18.4369, 44.0823) (-18.3651, 44.0902) (-18.3262, 44.0945) knots 0 0 0 0 0.009906 0.021634 0.021634 0.021634 0.021634
  spline S153 degree 3 poles (-18.3262, 44.0945) (-18.2793, 44.0981) (-18.1758, 44.106) (-18.0721, 44.1065) (-18.0154, 44.1068) knots 0 0 0 0 0.014107 0.03111 0.03111 0.03111 0.03111
  spline S154 degree 3 poles (-18.0154, 44.1068) (-17.9566, 44.1065) (-17.8488, 44.106) (-17.7413, 44.0981) (-17.6923, 44.0945) knots 0 0 0 0 0.017618 0.032339 0.032339 0.032339 0.032339
  spline S155 degree 3 poles (-17.6923, 44.0945) (-17.6518, 44.0903) (-17.578, 44.0826) (-17.5063, 44.0633) (-17.4738, 44.0545) knots 0 0 0 0 0.012185 0.02224 0.02224 0.02224 0.02224
  spline S156 degree 3 poles (-17.4738, 44.0545) (-17.4476, 44.045) (-17.3988, 44.0274) (-17.3617, 43.9912) (-17.3446, 43.9745) knots 0 0 0 0 0.008263 0.015355 0.015355 0.015355 0.015355
  spline S157 degree 3 poles (-17.3446, 43.9745) (-17.3308, 43.9548) (-17.301, 43.9122) (-17.2853, 43.8626) (-17.2769, 43.836) knots 0 0 0 0 0.007192 0.015493 0.015493 0.015493 0.015493
  line L47 (-17.2769, 43.836) -> (-15.6092, 37.8237)
  line L48 (-15.6092, 37.8237) -> (-15.5969, 37.8237)
  line L49 (-15.5969, 37.8237) -> (-14.0585, 43.836)
  spline S158 degree 3 poles (-14.0585, 43.836) (-14.0518, 43.8627) (-14.0394, 43.9125) (-14.0104, 43.9548) (-13.9969, 43.9745) knots 0 0 0 0 0.00815 0.015261 0.015261 0.015261 0.015261
  spline S159 degree 3 poles (-13.9969, 43.9745) (-13.9803, 43.9912) (-13.9451, 44.0265) (-13.8985, 44.0448) (-13.8738, 44.0545) knots 0 0 0 0 0.006976 0.01482 0.01482 0.01482 0.01482
  spline S160 degree 3 poles (-13.8738, 44.0545) (-13.8435, 44.0633) (-13.776, 44.0827) (-13.7061, 44.0903) (-13.6677, 44.0945) knots 0 0 0 0 0.009459 0.021034 0.021034 0.021034 0.021034
  spline S161 degree 3 poles (-13.6677, 44.0945) (-13.6198, 44.0981) (-13.5122, 44.1061) (-13.4044, 44.1066) (-13.3446, 44.1068) knots 0 0 0 0 0.014414 0.03234 0.03234 0.03234 0.03234
  spline S162 degree 3 poles (-13.3446, 44.1068) (-13.2825, 44.1065) (-13.1696, 44.106) (-13.0569, 44.0981) (-13.0062, 44.0945) knots 0 0 0 0 0.018618 0.033877 0.033877 0.033877 0.033877
  spline S163 degree 3 poles (-13.0062, 44.0945) (-12.9649, 44.0903) (-12.89, 44.0827) (-12.8173, 44.0633) (-12.7846, 44.0545) knots 0 0 0 0 0.012413 0.022544 0.022544 0.022544 0.022544
  spline S164 degree 3 poles (-12.7846, 44.0545) (-12.7582, 44.0449) (-12.7087, 44.027) (-12.6702, 43.9912) (-12.6523, 43.9745) knots 0 0 0 0 0.008334 0.015602 0.015602 0.015602 0.015602
  spline S165 degree 3 poles (-12.6523, 43.9745) (-12.6379, 43.9549) (-12.6073, 43.9131) (-12.5945, 43.8627) (-12.5877, 43.836) knots 0 0 0 0 0.007233 0.015407 0.015407 0.015407 0.015407
  line L50 (-12.5877, 43.836) -> (-10.4831, 36.4822)
  spline S166 degree 3 poles (-10.4831, 36.4822) (-10.4724, 36.4404) (-10.4537, 36.3674) (-10.4462, 36.2926) (-10.4431, 36.2607) knots 0 0 0 0 0.012932 0.02254 0.02254 0.02254 0.02254
  spline S167 degree 3 poles (-10.4431, 36.2607) (-10.4439, 36.2359) (-10.4455, 36.1888) (-10.4772, 36.1541) (-10.4923, 36.1376) knots 0 0 0 0 0.007158 0.013651 0.013651 0.013651 0.013651
  spline S168 degree 3 poles (-10.4923, 36.1376) (-10.5146, 36.1243) (-10.5667, 36.0934) (-10.627, 36.0863) (-10.6615, 36.0822) knots 0 0 0 0 0.007707 0.01798 0.01798 0.01798 0.01798
  spline S169 degree 3 poles (-10.6615, 36.0822) (-10.7072, 36.0786) (-10.8116, 36.0704) (-10.9164, 36.0701) (-10.9754, 36.0699) knots 0 0 0 0 0.013723 0.031418 0.031418 0.031418 0.031418
  spline S170 degree 3 poles (-10.9754, 36.0699) (-11.0323, 36.07) (-11.1329, 36.0703) (-11.2333, 36.0764) (-11.2769, 36.0791) knots 0 0 0 0 0.017078 0.030174 0.030174 0.030174 0.030174
  spline S171 degree 3 poles (-11.2769, 36.0791) (-11.3098, 36.0821) (-11.3675, 36.0874) (-11.4225, 36.1053) (-11.4462, 36.113) knots 0 0 0 0 0.009856 0.017306 0.017306 0.017306 0.017306
  spline S172 degree 3 poles (-11.4462, 36.113) (-11.4638, 36.1213) (-11.4965, 36.1369) (-11.5168, 36.1668) (-11.5262, 36.1807) knots 0 0 0 0 0.005725 0.010651 0.010651 0.010651 0.010651
  spline S173 degree 3 poles (-11.5262, 36.1807) (-11.5331, 36.1969) (-11.5483, 36.2326) (-11.5559, 36.2707) (-11.56, 36.2914) knots 0 0 0 0 0.005285 0.01161 0.01161 0.01161 0.01161
  line L51 (-11.56, 36.2914) -> (-13.3508, 42.9622)
  line L52 (-13.3508, 42.9622) -> (-13.3569, 42.9622)
  line L53 (-13.3569, 42.9622) -> (-15.0554, 36.3037)
  spline S174 degree 3 poles (-15.0554, 36.3037) (-15.0616, 36.2827) (-15.0732, 36.2432) (-15.0925, 36.2068) (-15.1015, 36.1899) knots 0 0 0 0 0.006568 0.012313 0.012313 0.012313 0.012313
  spline S175 degree 3 poles (-15.1015, 36.1899) (-15.1127, 36.1752) (-15.1364, 36.1441) (-15.172, 36.1278) (-15.1908, 36.1191) knots 0 0 0 0 0.005449 0.011546 0.011546 0.011546 0.011546
  spline S176 degree 3 poles (-15.1908, 36.1191) (-15.2155, 36.1112) (-15.2726, 36.093) (-15.3323, 36.0861) (-15.3662, 36.0822) knots 0 0 0 0 0.007766 0.01796 0.01796 0.01796 0.01796
  spline S177 degree 3 poles (-15.3662, 36.0822) (-15.41, 36.0786) (-15.5093, 36.0705) (-15.6089, 36.0701) (-15.6646, 36.0699) knots 0 0 0 0 0.013186 0.029881 0.029881 0.029881 0.029881
  spline S178 degree 3 poles (-15.6646, 36.0699) (-15.7162, 36.0701) (-15.8077, 36.0704) (-15.8987, 36.0786) (-15.9385, 36.0822) knots 0 0 0 0 0.015465 0.027423 0.027423 0.027423 0.027423
  spline S179 degree 3 poles (-15.9385, 36.0822) (-15.9692, 36.0863) (-16.0247, 36.0936) (-16.0779, 36.1113) (-16.1015, 36.1191) knots 0 0 0 0 0.009282 0.016753 0.016753 0.016753 0.016753
  spline S180 degree 3 poles (-16.1015, 36.1191) (-16.1203, 36.1278) (-16.156, 36.1441) (-16.1796, 36.1752) (-16.1908, 36.1899) knots 0 0 0 0 0.006097 0.011546 0.011546 0.011546 0.011546
  spline S181 degree 3 poles (-16.1908, 36.1899) (-16.1998, 36.2068) (-16.2191, 36.2432) (-16.2307, 36.2827) (-16.2369, 36.3037) knots 0 0 0 0 0.005745 0.012313 0.012313 0.012313 0.012313
  line L54 (-16.2369, 36.3037) -> (-18.0646, 42.9622)
  line L55 (-18.0646, 42.9622) -> (-18.0769, 42.9622)
  line L56 (-18.0769, 42.9622) -> (-19.8308, 36.2976)
  spline S182 degree 3 poles (-19.8308, 36.2976) (-19.8367, 36.2783) (-19.8479, 36.242) (-19.8614, 36.2065) (-19.8677, 36.1899) knots 0 0 0 0 0.006057 0.011387 0.011387 0.011387 0.011387
  spline S183 degree 3 poles (-19.8677, 36.1899) (-19.8761, 36.1752) (-19.8942, 36.1436) (-19.9271, 36.1276) (-19.9446, 36.1191) knots 0 0 0 0 0.004972 0.010672 0.010672 0.010672 0.010672
  spline S184 degree 3 poles (-19.9446, 36.1191) (-19.968, 36.1112) (-20.0221, 36.0931) (-20.0787, 36.0861) (-20.1108, 36.0822) knots 0 0 0 0 0.007397 0.017059 0.017059 0.017059 0.017059
  spline S185 degree 3 poles (-20.1108, 36.0822) (-20.1525, 36.0786) (-20.2477, 36.0705) (-20.3433, 36.0701) (-20.3969, 36.0699) knots 0 0 0 0 0.012572 0.028652 0.028652 0.028652 0.028652
  spline S186 degree 3 poles (-20.3969, 36.0699) (-20.4521, 36.0701) (-20.5498, 36.0705) (-20.647, 36.0808) (-20.6892, 36.0853) knots 0 0 0 0 0.016543 0.029288 0.029288 0.029288 0.029288
  spline S187 degree 3 poles (-20.6892, 36.0853) (-20.7212, 36.0904) (-20.7776, 36.0994) (-20.8254, 36.1303) (-20.8462, 36.1437) knots 0 0 0 0 0.009571 0.016908 0.016908 0.016908 0.016908
  spline S188 degree 3 poles (-20.8462, 36.1437) (-20.8603, 36.1603) (-20.8905, 36.1956) (-20.8917, 36.2422) (-20.8923, 36.2668) knots 0 0 0 0 0.006359 0.013506 0.013506 0.013506 0.013506
  spline S189 degree 3 poles (-20.8923, 36.2668) (-20.8895, 36.2987) (-20.883, 36.3732) (-20.8674, 36.4465) (-20.8585, 36.4884) knots 0 0 0 0 0.009591 0.02243 0.02243 0.02243 0.02243
  line L57 (-20.8585, 36.4884) -> (-18.7477, 43.836)
  spline S190 degree 3 poles (7.4246, 55.3807) (7.4323, 55.6883) (7.4469, 56.2771) (7.5859, 56.8491) (7.6523, 57.1222) knots 0 0 0 0 0.092022 0.176083 0.176083 0.176083 0.176083
  spline S191 degree 3 poles (7.6523, 57.1222) (7.7348, 57.3677) (7.8945, 57.8426) (8.1897, 58.2469) (8.3323, 58.4422) knots 0 0 0 0 0.077178 0.149269 0.149269 0.149269 0.149269
  spline S192 degree 3 poles (8.3323, 58.4422) (8.4941, 58.6138) (8.8218, 58.9614) (9.2506, 59.1723) (9.4677, 59.2791) knots 0 0 0 0 0.070141 0.142072 0.142072 0.142072 0.142072
  spline S193 degree 3 poles (9.4677, 59.2791) (9.7121, 59.3643) (10.2278, 59.5441) (10.7741, 59.562) (11.0615, 59.5714) knots 0 0 0 0 0.077179 0.162876 0.162876 0.162876 0.162876
  spline S194 degree 3 poles (11.0615, 59.5714) (11.3433, 59.5633) (11.8744, 59.5479) (12.3786, 59.3817) (12.6154, 59.3037) knots 0 0 0 0 0.084036 0.158412 0.158412 0.158412 0.158412
  spline S195 degree 3 poles (12.6154, 59.3037) (12.8232, 59.2058) (13.2323, 59.0129) (13.5447, 58.6861) (13.6985, 58.5253) knots 0 0 0 0 0.068267 0.1344 0.1344 0.1344 0.1344
  spline S196 degree 3 poles (13.6985, 58.5253) (13.8333, 58.3398) (14.1148, 57.9524) (14.2598, 57.4957) (14.3354, 57.2576) knots 0 0 0 0 0.068317 0.142693 0.142693 0.142693 0.142693
  spline S197 degree 3 poles (14.3354, 57.2576) (14.3964, 56.9874) (14.5257, 56.4143) (14.5381, 55.8266) (14.5446, 55.516) knots 0 0 0 0 0.082884 0.1758 0.1758 0.1758 0.1758
  spline S198 degree 3 poles (14.5446, 55.516) (14.5368, 55.215) (14.5217, 54.6365) (14.3833, 54.0748) (14.3169, 53.8053) knots 0 0 0 0 0.090026 0.173033 0.173033 0.173033 0.173033
  spline S199 degree 3 poles (14.3169, 53.8053) (14.2342, 53.5617) (14.0741, 53.0902) (13.7773, 52.6907) (13.6338, 52.4976) knots 0 0 0 0 0.076635 0.148341 0.148341 0.148341 0.148341
  spline S200 degree 3 poles (13.6338, 52.4976) (13.4711, 52.3277) (13.141, 51.9833) (12.7125, 51.7733) (12.4954, 51.6668) knots 0 0 0 0 0.069994 0.141916 0.141916 0.141916 0.141916
  spline S201 degree 3 poles (12.4954, 51.6668) (12.251, 51.5816) (11.7353, 51.4018) (11.189, 51.3839) (10.9015, 51.3745) knots 0 0 0 0 0.077179 0.162876 0.162876 0.162876 0.162876
  spline S202 degree 3 poles (10.9015, 51.3745) (10.6247, 51.3828) (10.101, 51.3984) (9.6037, 51.562) (9.3692, 51.6391) knots 0 0 0 0 0.082573 0.156221 0.156221 0.156221 0.156221
  spline S203 degree 3 poles (9.3692, 51.6391) (9.1619, 51.7363) (8.7529, 51.9279) (8.4383, 52.2517) (8.2831, 52.4114) knots 0 0 0 0 0.068052 0.134259 0.134259 0.134259 0.134259
  spline S204 degree 3 poles (8.2831, 52.4114) (8.1464, 52.5952) (7.862, 52.9778) (7.7139, 53.4312) (7.6369, 53.6668) knots 0 0 0 0 0.068228 0.142024 0.142024 0.142024 0.142024
  spline S205 degree 3 poles (7.6369, 53.6668) (7.575, 53.9331) (7.4441, 54.4967) (7.4313, 55.0754) (7.4246, 55.3807) knots 0 0 0 0 0.081796 0.173104 0.173104 0.173104 0.173104
  spline S206 degree 3 poles (8.5446, 55.4545) (8.5489, 55.2363) (8.5572, 54.8137) (8.6295, 54.3974) (8.6645, 54.196) knots 0 0 0 0 0.065376 0.126579 0.126579 0.126579 0.126579
  spline S207 degree 3 poles (8.6645, 54.196) (8.7092, 54.0116) (8.7952, 53.6563) (8.9767, 53.3393) (9.064, 53.1868) knots 0 0 0 0 0.05661 0.109028 0.109028 0.109028 0.109028
  spline S208 degree 3 poles (9.064, 53.1868) (9.1656, 53.0518) (9.3702, 52.7798) (9.6632, 52.6064) (9.8107, 52.5191) knots 0 0 0 0 0.050159 0.101042 0.101042 0.101042 0.101042
  spline S209 degree 3 poles (9.8107, 52.5191) (9.9827, 52.4492) (10.3526, 52.2989) (10.7523, 52.286) (10.9662, 52.2791) knots 0 0 0 0 0.055253 0.118841 0.118841 0.118841 0.118841
  spline S210 degree 3 poles (10.9662, 52.2791) (11.1804, 52.2867) (11.5823, 52.301) (11.95, 52.4623) (12.1216, 52.5376) knots 0 0 0 0 0.063634 0.119357 0.119357 0.119357 0.119357
  spline S211 degree 3 poles (12.1216, 52.5376) (12.2697, 52.6304) (12.5639, 52.8149) (12.7756, 53.0901) (12.8807, 53.2268) knots 0 0 0 0 0.051973 0.103258 0.103258 0.103258 0.103258
  spline S212 degree 3 poles (12.8807, 53.2268) (12.9717, 53.3793) (13.1597, 53.6943) (13.2513, 54.0496) (13.2986, 54.233) knots 0 0 0 0 0.052985 0.109449 0.109449 0.109449 0.109449
  spline S213 degree 3 poles (13.2986, 54.233) (13.3354, 54.4291) (13.4102, 54.8287) (13.4198, 55.2352) (13.4246, 55.4422) knots 0 0 0 0 0.059752 0.121755 0.121755 0.121755 0.121755
  spline S214 degree 3 poles (13.4246, 55.4422) (13.4205, 55.6673) (13.4127, 56.101) (13.3419, 56.5288) (13.3078, 56.7345) knots 0 0 0 0 0.067448 0.129911 0.129911 0.129911 0.129911
  spline S215 degree 3 poles (13.3078, 56.7345) (13.2644, 56.9213) (13.181, 57.2794) (13.0008, 57.5997) (12.9145, 57.753) knots 0 0 0 0 0.057189 0.109673 0.109673 0.109673 0.109673
  spline S216 degree 3 poles (12.9145, 57.753) (12.814, 57.8878) (12.6119, 58.1591) (12.3204, 58.3311) (12.1738, 58.4176) knots 0 0 0 0 0.049902 0.100403 0.100403 0.100403 0.100403
  spline S217 degree 3 poles (12.1738, 58.4176) (12.0015, 58.4866) (11.6283, 58.636) (11.2259, 58.648) (11.0092, 58.6545) knots 0 0 0 0 0.055253 0.11967 0.11967 0.11967 0.11967
  spline S218 degree 3 poles (11.0092, 58.6545) (10.793, 58.6469) (10.3872, 58.6326) (10.0152, 58.4713) (9.8414, 58.396) knots 0 0 0 0 0.064246 0.120547 0.120547 0.120547 0.120547
  spline S219 degree 3 poles (9.8414, 58.396) (9.6917, 58.3028) (9.394, 58.1175) (9.1838, 57.837) (9.0793, 57.6976) knots 0 0 0 0 0.052421 0.104181 0.104181 0.104181 0.104181
  spline S220 degree 3 poles (9.0793, 57.6976) (8.9894, 57.5424) (8.804, 57.2226) (8.7139, 56.8638) (8.6675, 56.6791) knots 0 0 0 0 0.053521 0.110336 0.110336 0.110336 0.110336
  spline S221 degree 3 poles (8.6675, 56.6791) (8.6317, 56.4812) (8.5584, 56.0763) (8.5493, 55.6648) (8.5446, 55.4545) knots 0 0 0 0 0.060248 0.123246 0.123246 0.123246 0.123246
  spline S222 degree 3 poles (2.6862, 59.2699) (2.6948, 59.2911) (2.7114, 59.3317) (2.7401, 59.3648) (2.7538, 59.3807) knots 0 0 0 0 0.006813 0.01306 0.01306 0.01306 0.01306
  spline S223 degree 3 poles (2.7538, 59.3807) (2.7704, 59.3945) (2.8062, 59.4244) (2.8502, 59.44) (2.8738, 59.4484) knots 0 0 0 0 0.006431 0.013875 0.013875 0.013875 0.013875
  spline S224 degree 3 poles (2.8738, 59.4484) (2.9029, 59.456) (2.9676, 59.4731) (3.0342, 59.479) (3.0708, 59.4822) knots 0 0 0 0 0.009012 0.020013 0.020013 0.020013 0.020013
  spline S225 degree 3 poles (3.0708, 59.4822) (3.1156, 59.4849) (3.215, 59.4908) (3.3146, 59.4912) (3.3692, 59.4914) knots 0 0 0 0 0.013479 0.029865 0.029865 0.029865 0.029865
  spline S226 degree 3 poles (3.3692, 59.4914) (3.4115, 59.4913) (3.4905, 59.4912) (3.5695, 59.4893) (3.6062, 59.4884) knots 0 0 0 0 0.012693 0.023695 0.023695 0.023695 0.023695
  spline S227 degree 3 poles (3.6062, 59.4884) (3.6377, 59.4871) (3.6965, 59.4848) (3.7547, 59.4767) (3.7815, 59.473) knots 0 0 0 0 0.009477 0.017615 0.017615 0.017615 0.017615
  spline S228 degree 3 poles (3.7815, 59.473) (3.8044, 59.469) (3.8469, 59.4616) (3.8885, 59.4504) (3.9077, 59.4453) knots 0 0 0 0 0.00697 0.012921 0.012921 0.012921 0.012921
  spline S229 degree 3 poles (3.9077, 59.4453) (3.9241, 59.44) (3.9554, 59.43) (3.9836, 59.4132) (3.9969, 59.4053) knots 0 0 0 0 0.005159 0.009806 0.009806 0.009806 0.009806
  spline S230 degree 3 poles (3.9969, 59.4053) (4.0085, 59.3968) (4.031, 59.3804) (4.0474, 59.3578) (4.0554, 59.3468) knots 0 0 0 0 0.004265 0.008313 0.008313 0.008313 0.008313
  spline S231 degree 3 poles (4.0554, 59.3468) (4.0626, 59.3344) (4.0781, 59.3078) (4.0894, 59.2791) (4.0954, 59.2637) knots 0 0 0 0 0.004304 0.009233 0.009233 0.009233 0.009233
  line L58 (4.0954, 59.2637) -> (6.6985, 51.8668)
  spline S232 degree 3 poles (6.6985, 51.8668) (6.7128, 51.8264) (6.738, 51.7554) (6.7469, 51.6806) (6.7508, 51.6484) knots 0 0 0 0 0.012798 0.022524 0.022524 0.022524 0.022524
  spline S233 degree 3 poles (6.7508, 51.6484) (6.7499, 51.6227) (6.7481, 51.5739) (6.7145, 51.5389) (6.6985, 51.5222) knots 0 0 0 0 0.007398 0.014091 0.014091 0.014091 0.014091
  spline S234 degree 3 poles (6.6985, 51.5222) (6.6748, 51.509) (6.6195, 51.4779) (6.5563, 51.4709) (6.52, 51.4668) knots 0 0 0 0 0.00805 0.018852 0.018852 0.018852 0.018852